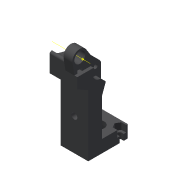
# Autodesk Inventor part: linact_knuckle
Saved by Autodesk Inventor 2014 (Build 180170000, 170)
## iProperties
Created: 2015-04-19
Part Number: linact_knuckle
Material: Generic
Document SubType Name: Modeling
Designer: Martin
Density: 1 g/cm^3
Appearance: Default
Author: Martin
Autodesk Inventor part; units mm, degrees
sketch "Sketch1" plane through (0, 0, 0) normal (0, 0, 1) x (1, 0, 0)
  circle A0 centre (-0.1255, -7.0715) radius 1 projected
  circle A1 centre (-5.6953, -4.5842) radius 1 projected
  circle A2 centre (5.8715, 6.6985) radius 1 projected
  line L0 (-4.1255, -10.2715) -> (3.8745, -10.2715) projected
  line L1 (-10.5, 0) -> (10.5, 0) projected
  line L2 (0, -14.2715) -> (0, 13.7285) projected
  line L3 (-7.5, -10.2715) -> (7.5, -10.2715)
  line L4 (7.5, -10.2715) -> (7.5, 9.7285)
  line L5 (7.5, 9.7285) -> (-7.5, 9.7285)
  line L6 (-7.5, 9.7285) -> (-7.5, -10.2715)
  line L7 (-7.5, -10.2715) -> (7.5, 9.7285) construction
  line L8 (7.5, -10.2715) -> (-7.5, 9.7285) construction
  circle A3 centre (-0.1255, 1.9285) radius 5.25 projected
  circle A4 centre (-0.1255, 1.9285) radius 5.5
  line L9 (7.5, 7.6985) -> (5.8715, 7.6985)
  line L10 (7.5, 5.6985) -> (5.8715, 5.6985)
  arc A5 (5.8715, 7.6985) -> (5.8715, 5.6985) centre (5.8715, 6.6985) ccw
  line L11 (-5.6953, -5.5842) -> (-7.5, -5.5842)
  line L12 (-5.6953, -3.5842) -> (-7.5, -3.5842)
  arc A6 (-5.6953, -5.5842) -> (-5.6953, -3.5842) centre (-5.6953, -4.5842) ccw
  point P0 (0, 0)
  point P1 (0, -0.2715)
  dimension "d0" = 11
  dimension "d4" = 15
  dimension "d5" = 20
  constraints: 20 end point, 8 point on circle, 8 tangent, 4 parallel, 4 point on line, 3 centre point, 3 midpoint, 3 perpendicular, 1 coincident, 1 collinear, 1 concentric, 1 horizontal
  measures "d0" diameter of A4
  measures "d4" distance of L4.end L5.end
  measures "d5" distance between parallel lines of L0 L5
extrude "ext_base" add sketch "Sketch1" along normal blind 4.3 contours A0 L2 | A0 L2 A4 L1 L4 L3 L0 | L2 A0 | A0 L2 L0 L3 L6 L11 A1 L12 L1 A4 | L1 L6 L5 L2 A4 | A4 L2 L5 L4 L9 A2 L10 L1
sketch "Sketch2" plane through (0, 0, 0) normal (0, 0, -1) x (-1, 0, 0)
  circle A0 centre (0.1255, -7.0715) radius 1 projected
  point P0 (0, 0)
extrude "ext_cut_dowel" cut sketch "Sketch2" against normal blind 1
sketch "Sketch3" plane through (0, 0, 4.3) normal (0, 0, 1) x (1, 0, 0)
  circle A0 centre (-0.1255, 1.9285) radius 5.5 projected
  line L0 (-7.5, -10.2715) -> (7.5, -10.2715) projected
  line L1 (7.5, -10.2715) -> (7.5, 5.6985) projected
  line L2 (7.5, 5.6985) -> (5.8715, 5.6985) projected
  arc A1 (5.8715, 7.6985) -> (5.8715, 5.6985) centre (5.8715, 6.6985) ccw projected
  line L3 (5.8715, 7.6985) -> (7.5, 7.6985) projected
  line L4 (7.5, 7.6985) -> (7.5, 9.7285) projected
  line L5 (7.5, 9.7285) -> (-7.5, 9.7285) projected
  line L6 (-7.5, 9.7285) -> (-7.5, -3.5842) projected
  line L7 (-7.5, -3.5842) -> (-5.6953, -3.5842) projected
  arc A2 (-5.6953, -5.5842) -> (-5.6953, -3.5842) centre (-5.6953, -4.5842) ccw projected
  line L8 (-5.6953, -5.5842) -> (-7.5, -5.5842) projected
  line L9 (-7.5, -5.5842) -> (-7.5, -10.2715) projected
  circle A3 centre (-0.1255, 1.9285) radius 3
  line L10 (-7.5, -3.5842) -> (-7.5, -5.5842)
  line L11 (7.5, 7.6985) -> (7.5, 5.6985)
  point P0 (0, 0)
  dimension "d10" = 6
  constraints: 4 end point, 2 collinear, 1 centre point, 1 coincident
  measures "d10" diameter of A3
extrude "ext_bearingstop" add sketch "Sketch3" along normal blind 2 contours A0 | L9 L8 A2 L7 L6 L5 L4 L3 A1 L2 L1 L0 | L10 L7 A2 L8 | L2 A1 L3 L11
sketch "Sketch4" plane through (0, 0, 0) normal (1, 0, 0) x (0, 1, 0)
  line L0 (0, -9.9126) -> (0, 59.4755) projected
  line L1 (-1.0715, 6.3) -> (4.9285, 6.3) projected
  line L2 (-10.2715, 6.3) -> (9.7285, 6.3) projected
  line L3 (9.7285, 6.3) -> (-10.2715, 6.3) projected
  line L4 (-1.0715, 6.3) -> (4.9285, 6.3) projected
  line L5 (1.9285, 6.3) -> (1.9285, 14.2197) construction
  line L6 (-10.2715, 6.3) -> (-1.2715, 6.3)
  line L7 (-1.2715, 6.3) -> (-1.2715, 34.3)
  line L8 (-1.2715, 34.3) -> (-10.2715, 34.3)
  line L9 (-10.2715, 34.3) -> (-10.2715, 6.3)
  line L10 (-10.2715, 6.3) -> (9.7285, 6.3) projected
  line L11 (-1.2715, 13.3) -> (5.7285, 6.3)
  line L12 (5.7285, 6.3) -> (-1.2715, 6.3)
  circle A0 centre (-4.0215, 37.05) radius 1
  circle A1 centre (-13.0215, 46.05) radius 1
  circle A2 centre (-13.0215, 46.05) radius 2.75 construction
  circle A3 centre (-4.0215, 37.05) radius 2.75 construction
  line L13 (-4.0215, 37.05) -> (-13.0215, 37.05) construction
  line L14 (-13.0215, 37.05) -> (-13.0215, 46.05) construction
  line L15 (-1.2715, 34.3) -> (-1.2715, 37.05)
  line L16 (-15.7715, 46.05) -> (-15.7715, 34.3)
  line L17 (-15.7715, 34.3) -> (-10.2715, 31.1246)
  line L18 (-15.7715, 34.3) -> (-10.2715, 34.3) construction
  line L19 (-2.0769, 38.9945) -> (-11.0769, 47.9945)
  arc A4 (-1.2715, 37.05) -> (-2.0769, 38.9945) centre (-4.0215, 37.05) ccw
  arc A5 (-11.0769, 47.9945) -> (-15.7715, 46.05) centre (-13.0215, 46.05) ccw
  point P0 (0, 0)
  point P1 (5.6985, 6)
  point P2 (5.6985, 6)
  point P3 (-3.5842, 6)
  point P4 (-3.5842, 6)
  point P5 (-5.5842, 6)
  point P6 (-5.5842, 6)
  dimension "d13" = 9
  dimension "d17" = 3.2
  dimension "d21" = 45
  dimension "d22" = 7
  dimension "d37" = 28
  dimension "d38" = 2
  dimension "d39" = 5.5
  dimension "d40" = 9
  dimension "d41" = 30
  constraints: 28 end point, 8 point on circle, 7 tangent, 6 centre point, 5 parallel, 4 perpendicular, 3 equal radius, 2 coincident, 2 horizontal, 2 point on line, 1 midpoint, 1 vertical, 2 other
  measures "d13" distance between parallel lines of L9 L7
  measures "d17" distance between parallel lines of L7 L5
  measures "d21" angle of L7 L11
  measures "d22" distance of L11.end L6.end
  measures "d37" distance of L8.end L2.start
  measures "d38" diameter of A1
  measures "d39" diameter of A2
  measures "d40" distance of L13.end L14.end
  measures "d41" angle of L18 L17
extrude "ext_knuckle_column" add sketch "Sketch4" along normal up to surface (15 mm away) from surface at -7.5 contours L7 L2 L9 L8 | L8 L9 L17 L16 A5 L19 A4 L15
ref_plane "plane_basenuts" through (0, 0, 3) normal (0, 0, 1) x (1, 0, 0)
sketch "Sketch8" plane through (0, 0, 3) normal (0, 0, 1) x (1, 0, 0)
  arc A0 (5.8715, 7.6985) -> (5.8715, 5.6985) centre (5.8715, 6.6985) ccw
  arc A1 (-5.6953, -5.5842) -> (-5.6953, -3.5842) centre (-5.6953, -4.5842) ccw
  line L0 (-5.6953, -5.5842) -> (-7, -5.5842)
  line L1 (-7, -5.5842) -> (-7, -10.2715)
  line L2 (-7, -3.2715) -> (-7, -10.2715)
  line L3 (4.6014, 8.8985) -> (3.3312, 6.6985)
  line L4 (3.3312, 6.6985) -> (4.6014, 4.4985)
  line L5 (3.3312, 6.6985) -> (8.4119, 6.6985) construction
  line L6 (4.6014, 8.8985) -> (7.1417, 8.8985)
  line L7 (7.1417, 8.8985) -> (8.4119, 6.6985)
  line L8 (8.4119, 6.6985) -> (7.1417, 4.4985)
  line L9 (4.6014, 4.4985) -> (7.1417, 4.4985)
  line L10 (5.8715, 8.8985) -> (5.8715, 4.4985) construction
  line L11 (0, -14.2715) -> (0, 13.7285)
  line L12 (-8.2357, -4.5842) -> (-3.155, -4.5842) construction
  line L13 (-5.6953, -2.3842) -> (-5.6953, -6.7842) construction
  line L14 (-4.4252, -2.3842) -> (-6.9655, -2.3842)
  line L15 (-6.9655, -2.3842) -> (-8.2357, -4.5842)
  line L16 (-8.2357, -4.5842) -> (-6.9655, -6.7842)
  line L17 (-6.9655, -6.7842) -> (-4.4252, -6.7842)
  line L18 (-4.4252, -6.7842) -> (-3.155, -4.5842)
  line L19 (-4.4252, -2.3842) -> (-3.155, -4.5842)
  point P0 (0, 0)
  point P1 (-5.7187, -4.5372)
  dimension "d33" = 120
  dimension "d35" = 4.4
  dimension "d36" = 4.4
  constraints: 40 end point, 8 midpoint, 8 parallel, 4 equal length, 4 point on circle, 3 perpendicular, 2 centre point, 2 coincident
  measures "d33" angle of L4 L3
  measures "d35" distance between parallel lines of L9 L6
  measures "d36" distance between parallel lines of L17 L14
extrude "ext_cut_basenuts" cut sketch "Sketch8" along normal up to surface (3.3 mm away)
sketch "Sketch9" plane through (-7.5, -10.2715, 0) normal (-1, 0, 0) x (0, 0, 1)
  line L0 (46.05, -5.5) -> (34.3, -5.5) projected
  arc A0 (46.05, -5.5) -> (47.9945, -0.8055) centre (46.05, -2.75) ccw projected
  line L1 (38.9945, 8.1945) -> (47.9945, -0.8055) projected
  arc A1 (38.9945, 8.1945) -> (37.05, 9) centre (37.05, 6.25) ccw projected
  line L2 (6.3, 9) -> (37.05, 9) projected
  circle A2 centre (37.05, 6.25) radius 1 projected
  circle A3 centre (46.05, -2.75) radius 1 projected
  line L3 (30.4109, 9) -> (44.9109, -5.5)
  circle A4 centre (37.05, 6.25) radius 2.75 construction
  circle A5 centre (37.05, 6.25) radius 4
  circle A6 centre (46.05, -2.75) radius 4
  line L4 (43.2216, -5.5784) -> (43.1431, -5.5)
  line L5 (43.1431, -5.5) -> (43.1453, -5.5)
  point P0 (7, 7)
  point P1 (0, 10.2715)
  point P2 (6, 7)
  dimension "d45" = 8
  constraints: 6 end point, 3 centre point, 3 coincident, 3 point on line, 3 tangent, 2 parallel, 2 point on circle, 1 equal radius, 2 other
  measures "d45" diameter of A5
extrude "ext_cut_finger_right" cut sketch "Sketch9" against normal blind 2.5 contours L0 L3 A6 L1 A0 | L3 A5 L1 A6 | A5 L3 | L3 A5 L2 A1 L1 | L1 A1 L2 A5 | L3 L2 A5 | A2
sketch "Sketch11" plane through (-5, -10.2715, 0) normal (-1, 0, 0) x (0, 0, 1)
  arc A0 (46.05, -5.5) -> (47.9945, -0.8055) centre (46.05, -2.75) ccw projected
  line L0 (38.9945, 8.1945) -> (47.9945, -0.8055) projected
  arc A1 (38.9945, 8.1945) -> (37.05, 9) centre (37.05, 6.25) ccw projected
  circle A2 centre (46.05, -2.75) radius 1 projected
  circle A3 centre (37.05, 6.25) radius 1 projected
  circle A4 centre (46.05, -2.75) radius 2.75
  circle A5 centre (37.05, 6.25) radius 2.75
  line L1 (43.3, 3.8891) -> (43.3, -2.75) construction
  line L2 (40.7374, 6.4517) -> (43.3937, -3.4618)
  line L3 (40.7374, 6.4517) -> (47.9945, -0.8055)
  point P0 (0, 10.2715)
  dimension "d47" = 15
  constraints: 6 end point, 4 tangent, 3 point on circle, 2 centre point, 2 coincident, 2 point on line, 1 concentric, 1 vertical
  measures "d47" angle of L1 L2
extrude "ext_cut_linkattachment" cut sketch "Sketch11" against normal blind 5.5 contours A4 A0 | L2 L0 A4
fillet "Fillet1" radius 1 1 edges at (-2.25, -15.7715, 46.05)
ref_plane "Work Plane1" through (7.5, -13.0215, 46.05) normal (0, 1, 0) x (-1, 0, 0)
sketch "Sketch15" plane through (7.5, -13.0215, 46.05) normal (0, 1, 0) x (-1, 0, 0)
  line L0 (18, 0) -> (-3, 0) projected
  line L1 (7, -1) -> (7, 1) projected
  line L2 (7, -2.6563) -> (7, -5.3126) projected
  line L3 (7, -2.4322) -> (7, -2.6563) projected
  line L4 (7, -3.3166) -> (7, -2.4322) projected
  line L5 (7, -3.3166) -> (7, 0) projected
  line L6 (7, 1.9445) -> (7, 0) projected
  line L7 (7, -5.3126) -> (7, 1.9445) projected
  line L8 (0, -9) -> (0, -39.75) projected
  line L9 (0, -7.0555) -> (0, -9) projected
  line L10 (0, 1.9445) -> (0, -7.0555) projected
  line L11 (0, 0) -> (0, 1.9445) projected
  line L12 (0, -11.75) -> (0, 0) projected
  line L13 (0, -14.9254) -> (0, -11.75) projected
  line L14 (0, -46.05) -> (0, -14.9254) projected
  line L15 (0, -46.05) -> (0, -43.05) projected
  line L16 (0, -8) -> (0, -10) projected
  line L17 (0, 1) -> (0, -1) projected
  line L18 (7, 0) -> (7, 2.25)
  line L19 (7, 2.25) -> (6, 2.25)
  line L20 (6, 2.25) -> (6, 2.75)
  line L21 (6, 2.75) -> (2.5, 2.75)
  line L22 (2.5, 2.75) -> (2.5, 0)
  line L23 (2.5, 0) -> (7, 0)
  line L24 (0, -46.05) -> (0, -43.05) projected
  line L25 (0, -46.05) -> (0, -39.75) projected
  line L26 (0, -39.75) -> (0, -43.05) projected
  line L27 (0, -43.05) -> (0, -39.75) projected
  point P0 (7.5, -46.05)
  dimension "d66" = 2.25
  dimension "d67" = 2.75
  dimension "d68" = 1
  dimension "d69" = 3.5
  constraints: 12 end point, 2 parallel, 2 perpendicular, 2 point on line, 1 collinear
  measures "d66" distance between parallel lines of L23 L19
  measures "d67" distance between parallel lines of L0 L21
  measures "d68" distance of L18.end L19.end
  measures "d69" distance of L20.end L21.end
revolve "rev_squarepot_shaft" cut sketch "Sketch15" angle 360 about axis through (0, -13.0215, 46.05) along (1, 0, 0)
sketch "Sketch16" plane through (7.5, -10.2715, 0) normal (1, 0, 0) x (0, 0, -1)
  circle A0 centre (-46.05, -2.75) radius 1 projected
  line L0 (-39.55, -8.25) -> (-52.55, -8.25)
  line L1 (-52.55, -8.25) -> (-52.55, 2.75)
  line L2 (-52.55, 2.75) -> (-39.55, 2.75)
  line L3 (-39.55, 2.75) -> (-39.55, -8.25)
  line L4 (-39.55, -8.25) -> (-52.55, 2.75) construction
  line L5 (-52.55, -8.25) -> (-39.55, 2.75) construction
  point P0 (0, 10.2715)
  dimension "d71" = 13
  dimension "d72" = 11
  constraints: 12 end point, 2 midpoint, 2 parallel, 1 horizontal, 1 perpendicular
  measures "d71" distance of L1.end L2.end
  measures "d72" distance of L0.end L1.end
extrude "ext_squarepot_body" cut sketch "Sketch16" against normal up to surface (2.5 mm away)
sketch "Sketch17" plane through (7.5, -10.2715, 0) normal (1, 0, 0) x (0, 0, -1)
  line L0 (-37.05, 9) -> (-6.3, 9) projected
  arc A0 (-37.05, 9) -> (-38.9945, 8.1945) centre (-37.05, 6.25) ccw projected
  line L1 (-44.4391, 2.75) -> (-38.9945, 8.1945) projected
  circle A1 centre (-37.05, 6.25) radius 1 projected
  line L2 (-33.0515, 6.3594) -> (-30.4109, 9) projected
  arc A2 (-37.1594, 2.2515) -> (-33.0515, 6.3594) centre (-37.05, 6.25) ccw projected
  line L3 (-43.7137, -4.3028) -> (-37.1594, 2.2515) projected
  circle A3 centre (-37.05, 6.25) radius 4
  line L4 (-41.0485, 6.1406) -> (-44.4391, 2.75)
  line L5 (-44.4391, 2.75) -> (-35.1135, 2.75)
  line L6 (-34.1453, 9) -> (-30.4109, 9)
  line L7 (-30.4109, 9) -> (-33.0515, 6.3594)
  point P0 (0, 10.2715)
  constraints: 8 end point, 4 point on circle, 3 point on line, 1 centre point, 1 coincident, 1 concentric, 1 parallel
extrude "ext_cut_finger_left_2" cut sketch "Sketch17" against normal blind 2.5 contours L0 A3 A2 L5 L1 A0 | L0 L2 A3 | A3 L5 L1 | L5 A2 A3 | A1
sketch "Sketch18" plane through (5, -15.7715, 46.05) normal (1, 0, 0) x (0, 0, -1)
  circle A0 centre (0, 2.75) radius 3.75
  line L0 (1.6109, 8.25) -> (-2.0317, 5.9019)
  line L1 (0.5972, -0.9521) -> (6.5, 0)
  arc A1 (0, 0) -> (-1.9445, 4.6945) centre (0, 2.75) ccw projected
  line L2 (6.5, 0) -> (0, 0) projected
  line L3 (-1.9445, 4.6945) -> (7.0555, 13.6945) projected
  line L4 (1.6109, 8.25) -> (-0.1418, 6.4973)
  line L5 (6.5, 0) -> (2.5495, 0)
  circle A2 centre (0, 2.75) radius 2.75
  point P0 (46.05, 15.7715)
  dimension "d77" = 7.5
  constraints: 8 end point, 4 point on circle, 2 centre point, 2 coincident, 2 tangent, 1 collinear, 1 concentric, 1 point on line
  measures "d77" diameter of A0
extrude "ext_squarepot_reinforcement" add sketch "Sketch18" against normal up to surface (4.5 mm away) contours A0 L2 A1 L3 | L3 A2 L2 A0 | A0 L0 L3 | L2 L1 A0
sketch "Sketch24" plane through (7.5, -10.2715, 0) normal (1, 0, 0) x (0, 0, -1)
  line L0 (-30.4109, 9) -> (-6.3, 9) projected
  line L1 (-6.3, 7) -> (-25.255, 7)
  line L2 (-6.3, 9) -> (-30.4109, 9) projected
  line L3 (-6.3, 7) -> (-6.3, 9)
  line L4 (-30.75, 9) -> (-6.3, 9)
  arc A0 (-38.9865, 2.75) -> (-33.0515, 6.3594) centre (-37.05, 6.25) ccw projected
  line L5 (-25.255, 7) -> (-30.75, 9)
  circle A1 centre (-37.05, 6.25) radius 1 projected
  circle A2 centre (-37.05, 6.25) radius 1 projected
  point P0 (0, 10.2715)
  dimension "d99" = 2
  dimension "d104" = 160
  dimension "d105" = 6.3
  constraints: 8 end point, 1 collinear, 1 parallel, 1 perpendicular, 1 point on line
  measures "d99" distance of L0.end L1.start
  measures "d104" angle of L1 L5
  measures "d105" horizontal distance of L4.start A0.centre
extrude "ext_cut_linactrod_cutway" cut sketch "Sketch24" against normal through all contours L0 L3 L1 L5 L4
sketch "sk_fixation_nut" plane through (7.5, -3.2715, 25.255) normal (0, 1, 0) x (1, 0, 0)
  line L0 (-15, 0) -> (-15, 18.955) projected
  line L1 (0, 0) -> (-15, 0) projected
  line L2 (0, 18.955) -> (0, 0) projected
  line L3 (0, 18.955) -> (-11.4129, 18.955) projected
  line L4 (-7.5, 0) -> (-7.5, 18.955) construction
  line L5 (-15, 8.955) -> (0, 8.955) construction
  line L6 (-4.0359, 8.955) -> (-5.7679, 11.955)
  line L7 (-5.7679, 11.955) -> (-9.2321, 11.955)
  line L8 (-9.2321, 11.955) -> (-10.9641, 8.955)
  line L9 (-10.9641, 8.955) -> (-9.2321, 5.955)
  line L10 (-9.2321, 5.955) -> (-5.7679, 5.955)
  line L11 (-5.7679, 5.955) -> (-4.0359, 8.955)
  circle A0 centre (-7.5, 8.955) radius 1.5
  point P0 (-14, 19.955)
  point P1 (-10.9129, 19.955)
  point P2 (-7.5, 25.255)
  point P3 (-7.5, 11.955)
  point P4 (-7.5, 5.955)
  point P5 (-14, 18.955)
  dimension "d106" = 10
  dimension "d107" = 120
  dimension "d108" = 6
  dimension "d109" = 3
  constraints: 16 end point, 6 point on line, 5 equal length, 4 midpoint, 1 centre point, 1 parallel, 1 perpendicular, 1 vertical, 4 other
  measures "d107" angle of L11 L6
  measures "d108" distance between parallel lines of L10 L7
  measures "d109" diameter of A0
extrude "ext_cut_fixation_nut" [suppressed]
extrude "ext_cut_fixation_screw" cut sketch "sk_fixation_nut" against normal through all contours A0
sketch "Sketch26" plane through (5, -15.7715, 39.55) normal (1, 0, 0) x (0, 0, -1)
  line L0 (0, 8.25) -> (0, 0) projected
  circle A0 centre (-6.5, 2.75) radius 2.75 projected
  line L1 (-6.5, 2.75) -> (0, 2.75) construction
  line L2 (-1.4, 1.55) -> (0, 1.55)
  line L3 (0, 1.55) -> (0, 3.95)
  line L4 (0, 3.95) -> (-1.4, 3.95)
  line L5 (-1.4, 3.95) -> (-1.4, 1.55)
  line L6 (-1.4, 1.55) -> (0, 3.95) construction
  line L7 (0, 1.55) -> (-1.4, 3.95) construction
  point P0 (39.55, 15.7715)
  point P1 (-0.7, 2.75)
  dimension "d115" = 2.4
  dimension "d116" = 1.4
  constraints: 14 end point, 3 point on line, 2 midpoint, 2 parallel, 2 perpendicular, 1 horizontal
  measures "d115" distance of L4.end L2.start
  measures "d116" distance of L3.end L4.end
extrude "ext_cut_squarepot_tab" cut sketch "Sketch26" against normal blind 2 contours L0 L2 L5 L4
sketch "Sketch28" plane through (0.5, -10.2715, 0) normal (-1, 0, 0) x (0, 0, 1)
  arc A0 (45.4528, -6.4521) -> (48.0817, 0.4019) centre (46.05, -2.75) ccw projected
  circle A1 centre (46.05, -2.75) radius 2.75
  point P0 (0, 10.2715)
  point P1 (43.5005, -5.5)
  point P2 (46.1918, 0.9973)
  dimension "d130" = 5.5
  constraints: 1 centre point, 1 coincident
  measures "d130" diameter of A1
extrude "QFIX_ext_cut_potdiameter" cut sketch "Sketch28" against normal through all
ref_plane "plane_support_base" through (-7.5, -3.5842, 0) normal (-1, 0, 0) x (0, 0, 1)
sketch "sk_support" plane through (-7.5, -3.5842, 0) normal (-1, 0, 0) x (0, 0, 1)
  arc A0 (45.4528, -13.1394) -> (48.0817, -6.2854) centre (46.05, -9.4373) ccw projected
  line L0 (43.3937, -10.149) -> (40.7374, -0.2356) projected
  line L1 (43.7137, -10.9901) -> (37.1594, -4.4358) projected
  line L2 (33.0515, -0.3279) -> (30.5014, 2.2222) projected
  line L3 (30.75, 2.3127) -> (37.05, 2.3127) projected
  line L4 (31.8251, 2.3127) -> (44.7137, -10.5759)
  line L5 (44.7137, -10.5759) -> (44.7137, -13.1659)
  line L6 (44.7137, -13.1659) -> (45.9887, -13.1868)
  line L7 (48.0817, -6.2854) -> (39.4837, 2.3127)
  line L8 (39.4837, 2.3127) -> (31.8251, 2.3127)
  arc A1 (45.9887, -13.1868) -> (48.0817, -6.2854) centre (46.05, -9.4373) ccw
  line L9 (41.6778, 0.1186) -> (44.481, -10.3431)
  point P0 (0, 3.5842)
  point P1 (43.5005, -12.1873)
  point P2 (46.1918, -5.6899)
  dimension "d120" = 1
  dimension "d121" = 1
  dimension "d125" = 1
  constraints: 12 end point, 3 parallel, 3 point on circle, 3 point on line, 1 centre point, 1 collinear, 1 concentric, 1 perpendicular, 1 tangent
  measures "d120" distance from line of L5 L1.start
  measures "d121" distance between parallel lines of L4 L2
  measures "d125" distance between parallel lines of L9 L0
ref_plane "plane_support_top_1" through (-5.4, -10.2715, 0) normal (-1, 0, 0) x (0, 0, 1)
ref_plane "plane_support_top_2" through (0.1, -10.2715, 0) normal (-1, 0, 0) x (0, 0, 1)
extrude "PRINT_ext_support_1" [suppressed]
extrude "PRINT_ext_support_2" [suppressed]
equation "\"d0\" = linact_bearing_diameter"
equation "\"d4\" = model_column_thickness"
equation "\"d6\" = linact_bearing_thickness"
equation "\"d39\" = general_bore_smallersupport_diameter"
equation "\"d108\" = nut_m3_width_acrossflats"
equation "\"d109\" = screw_m3_bore_selfthreading"
equation "\"d120\" = print_support_xy_clearance"
equation "\"d121\" = print_support_xy_clearance"
equation "\"d125\" = print_support_xy_clearance"
equation "\"general_bore_smallersupport_diameter\" = 5.5"
equation "\"d123\" = print_support_z_clearance"
equation "\"d124\" = print_support_z_clearance"
equation "\"model_column_thickness\" = 15"
equation "\"model_fingerbase_thickness\" = 9"
equation "\"linact_bearing_diameter\" = 11"
equation "\"linact_bearing_thickness\" = 4.3"
equation "\"nut_m3_width_acrossflats\" = 6"
equation "\"screw_m3_bore_selfthreading\" = 3"
equation "\"print_support_xy_clearance\" = 1"
equation "\"print_support_z_clearance\" = 0.4"
body "Solid1"
